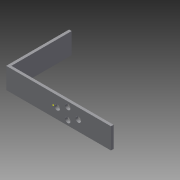
# Autodesk Inventor part: lBracketForLiftingBar
Saved by Autodesk Inventor 2015 (Build 190159000, 159)
## iProperties
Created: 2015-02-04
Part Number: lBracketForLiftingBar
Material: Generic
Document SubType Name: Modeling
Designer: Kingbob26
Density: 1 g/cm^3
Appearance: Default
Author: Kingbob26
Autodesk Inventor part; units mm, degrees
ref_plane "YZ Plane" through (0, 0, 0) normal (1, 0, 0) x (0, 1, 0)
ref_plane "XZ Plane" through (0, 0, 0) normal (0, 1, 0) x (-1, 0, 0)
ref_plane "XY Plane" through (0, 0, 0) normal (0, 0, 1) x (1, 0, 0)
sketch "Sketch1" plane through (0, 0, 0) normal (0, 0, 1) x (1, 0, 0)
  line L0 (57.15, 12.7) -> (-57.15, 12.7)
  line L1 (-57.15, 12.7) -> (-57.15, -12.7)
  line L2 (-57.15, -12.7) -> (57.15, -12.7)
  line L3 (57.15, -12.7) -> (57.15, 12.7)
  point P0 (0, 0)
  dimension "d0" = 114.3
  dimension "d1" = 25.4
  constraints: 8 end point, 2 parallel, 1 horizontal, 1 perpendicular
  measures "d0" distance of L2.end L1.end
  measures "d1" distance of L1.end L0.end
extrude "Extrusion1" add sketch "Sketch1" against normal blind 3.175
sketch "Sketch2" plane through (-57.15, -12.7, 0) normal (-1, 0, 0) x (0, 0, 1)
  line L0 (0, 25.4) -> (0, 0) projected
  line L1 (0, 25.4) -> (-3.175, 25.4) projected
  line L2 (-3.175, 0) -> (-3.175, 25.4) projected
  line L3 (0, 0) -> (-3.175, 0) projected
  point P0 (0, 12.7)
sketch "Sketch3" plane through (0, 0, 0) normal (0, 0, 1) x (1, 0, 0)
  line L0 (57.15, -12.7) -> (-57.15, -12.7) projected
  line L1 (-57.15, 12.7) -> (-53.975, 12.7)
  line L2 (-53.975, 12.7) -> (-53.975, -12.7)
  line L3 (-53.975, -12.7) -> (-57.15, -12.7)
  line L4 (-57.15, -12.7) -> (-57.15, 12.7)
  point P0 (0, 0)
  dimension "d4" = 3.175
  constraints: 8 end point, 2 parallel, 1 horizontal, 1 perpendicular, 1 point on line
  measures "d4" distance of L2.end L3.end
extrude "Extrusion2" cut sketch "Sketch2" against normal blind 3.175
extrude "Extrusion3" add sketch "Sketch3" against normal blind 76.2
sketch "Sketch4" plane through (0, 0, 0) normal (0, 0, 1) x (1, 0, 0)
  point P0 (0, 0)
sketch "Sketch5" plane through (0, 0, 0) normal (0, 0, 1) x (1, 0, 0)
  point P0 (0, 0)
sketch "Sketch6" plane through (57.15, -12.7, 0) normal (1, 0, 0) x (0, 0, -1)
  line L0 (0, 0) -> (0, 25.4) projected
  line L1 (0, 0) -> (3.175, 0) projected
  line L2 (3.175, 25.4) -> (3.175, 0) projected
  line L3 (0, 25.4) -> (3.175, 25.4) projected
  point P0 (0, 12.7)
extrude "Extrusion4" add sketch "Sketch6" along normal blind 12.7
sketch "Sketch7" plane through (0, 0, 0) normal (0, 0, 1) x (1, 0, 0)
  point P0 (0, 0)
sketch "Sketch8" plane through (0, 0, 0) normal (0, 0, 1) x (1, 0, 0)
  circle A0 centre (4.7498, 0) radius 3.2639
  point P0 (0, 0)
  dimension "d11" = 6.5278
  constraints: 1 centre point
  measures "d11" diameter of A0
extrude "Extrusion5" cut sketch "Sketch8" against normal blind 3.175
sketch "Sketch9" plane through (0, 0, 0) normal (0, 0, 1) x (1, 0, 0)
  circle A0 centre (30.1498, 0) radius 3.2639
  point P0 (0, 0)
  dimension "d14" = 6.5278
  constraints: 1 centre point
  measures "d14" diameter of A0
extrude "Extrusion6" cut sketch "Sketch9" against normal blind 3.175
sketch "Sketch10" plane through (0, 0, 0) normal (0, 0, 1) x (1, 0, 0)
  circle A0 centre (17.4498, 6.9088) radius 3.2639
  circle A1 centre (17.4498, -6.9088) radius 3.2639
  point P0 (0, 0)
  dimension "d17" = 6.5278
  dimension "d18" = 6.5278
  constraints: 2 centre point
  measures "d17" diameter of A0
  measures "d18" diameter of A1
extrude "Extrusion7" cut sketch "Sketch10" against normal blind 3.175
body "Solid1"
